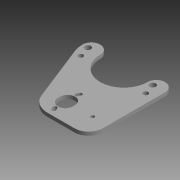
# Autodesk Inventor part: motor plate
Saved by Autodesk Inventor 2015 (Build 190159000, 159)
## iProperties
Created: 2015-08-29
Part Number: motor plate
Material: Generic
Description: insert part description/title
Document SubType Name: Modeling
Designer: francis
Density: 1 g/cm^3
Appearance: Default
Part Category: insert part category here and press enter to fill value
Author: francis
Autodesk Inventor part; units mm, degrees
ref_plane "YZ Plane" through (0, 0, 0) normal (1, 0, 0) x (0, 1, 0)
ref_plane "XZ Plane" through (0, 0, 0) normal (0, 1, 0) x (-1, 0, 0)
ref_plane "XY Plane" through (0, 0, 0) normal (0, 0, 1) x (1, 0, 0)
sketch "Sketch1" plane through (0, 0, 0) normal (0, 0, 1) x (1, 0, 0)
  line L0 (-15, 13.1624) -> (0, 13.1624) construction
  line L1 (-15, -13.1624) -> (-15, 13.1624) construction
  line L2 (0, -13.1624) -> (-15, -13.1624) construction
  line L3 (0, 13.1624) -> (0, -13.1624) construction
  circle A0 centre (15.5255, -58.6235) radius 1.2295 construction
  circle A1 centre (15.5255, -38.1235) radius 1.2295 construction
  circle A2 centre (37.6255, -48.3735) radius 1.2295 construction
  circle A3 centre (15.5255, -48.3735) radius 6 construction
  circle A4 centre (20, 0) radius 4 construction
  line L4 (40, 13.1624) -> (55, 13.1624) construction
  line L5 (40, -13.1624) -> (40, 13.1624) construction
  line L6 (55, -13.1624) -> (40, -13.1624) construction
  line L7 (55, 13.1624) -> (55, -13.1624) construction
  arc A5 (0, 0) -> (-15, 0) centre (-7.5, 0) ccw
  arc A6 (55, 0) -> (40, 0) centre (47.5, 0) ccw
  arc A7 (0, 0) -> (40, 0) centre (20, 0) ccw
  line L8 (53.51, -48.6) -> (3.95, -48.6) construction
  line L9 (15.5255, -64.6235) -> (43, -64.6235)
  line L10 (55, 0) -> (55, -52.6235)
  arc A8 (43, -64.6235) -> (55, -52.6235) centre (43, -52.6235) ccw
  line L11 (-0.0384, -53.0454) -> (-14.0792, -6.27)
  arc A9 (-0.0384, -53.0454) -> (15.5255, -64.6235) centre (15.5255, -48.3735) ccw
  arc A10 (-15, 0) -> (-14.0792, -6.27) centre (6.8084, 0) ccw
  circle A11 centre (37.6255, -48.3735) radius 1.5
  arc A12 (14.6588, -36.4849) -> (13.7101, -38.5318) centre (37.6255, -48.3735) ccw
  arc A13 (17.3231, -37.864) -> (16.4844, -39.6735) centre (37.6255, -48.3735) ccw
  arc A14 (16.4865, -57.0786) -> (17.3256, -58.8879) centre (37.6255, -48.3735) ccw construction
  arc A15 (13.7125, -58.2209) -> (14.6617, -60.2676) centre (37.6255, -48.3735) ccw
  arc A16 (14.6617, -60.2676) -> (17.3256, -58.8879) centre (15.9937, -59.5777) ccw
  arc A17 (16.4865, -57.0786) -> (13.7125, -58.2209) centre (15.0995, -57.6498) ccw
  arc A18 (13.7101, -38.5318) -> (16.4844, -39.6735) centre (15.0972, -39.1027) ccw
  arc A19 (17.3231, -37.864) -> (14.6588, -36.4849) centre (15.991, -37.1745) ccw
  arc A20 (15.0995, -57.6498) -> (15.9937, -59.5777) centre (37.6255, -48.3735) ccw construction
  arc A21 (15.991, -37.1745) -> (15.0972, -39.1027) centre (37.6255, -48.3735) ccw construction
  arc A22 (16.4865, -57.0786) -> (17.3256, -58.8879) centre (37.6255, -48.3735) ccw
  arc A23 (9.3039, -47.106) -> (9.3039, -49.641) centre (35.3706, -48.3735) ccw
  arc A24 (21.7892, -47.7131) -> (21.7892, -49.0339) centre (35.3706, -48.3735) ccw
  arc A25 (9.3039, -49.641) -> (21.7892, -49.0339) centre (15.5466, -49.3375) ccw
  arc A26 (21.7892, -47.7131) -> (9.3039, -47.106) centre (15.5466, -47.4095) ccw
  arc A27 (15.5466, -47.4095) -> (15.5466, -49.3375) centre (37.6255, -48.3735) ccw construction
  circle A28 centre (-7.5, -9) radius 1.7295
  circle A29 centre (47.5, -9) radius 1.7295
  circle A30 centre (47.5, -9) radius 2
  circle A31 centre (-7.5, -9) radius 2
  circle A32 centre (-10.5, 0) radius 2.067
  circle A33 centre (44.5, 0) radius 2.067
  circle A34 centre (-10.5, 0) radius 2.5
  circle A35 centre (44.5, 0) radius 2.5
extrude "Extrusion1" add sketch "Sketch1" along normal blind 3 contours A7 A6 L10 A8 L9 A9 L11 A10 A5
body "Solid1"
